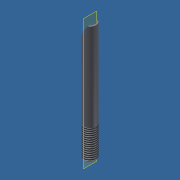
# Autodesk Inventor part: ESCAPAMENTO(16)
Saved by Autodesk Inventor 2012 SP1 (Build 160190100, 190)
## iProperties
Created: 2012-07-23
Part Number: ESCAPAMENTO(16)
Material: Carbon Steel
Document SubType Name: Modeling
Designer: bruno.silveira
Mass: 20.7136 g
Surface Area: 26.512 cm^2
Volume: 2.63197 cm^3
Density: 7.87 g/cm^3
Author: bruno.silveira
Autodesk Inventor part; units mm, degrees
ref_plane "YZ Plane" through (0, 0, 0) normal (1, 0, 0) x (0, 1, 0)
ref_plane "XZ Plane" through (0, 0, 0) normal (0, 1, 0) x (-1, 0, 0)
ref_plane "XY Plane" through (0, 0, 0) normal (0, 0, 1) x (1, 0, 0)
sketch "Sketch1" plane through (0, 0, 0) normal (0, 0, 1) x (1, 0, 0)
  circle A0 centre (0, 0) radius 3.9688
  dimension "d0" = 7.9375
  constraints: 1 centre point, 1 coincident
  measures "d0" diameter of A0
extrude "Extrusion1" add sketch "Sketch1" along normal blind 78
thread "Thread1" size "M8x1.25" class "6g" standard "ANSI Metric M Profile" length 20
sketch "Sketch2" plane through (0, 0, 78) normal (0, 0, 1) x (1, 0, 0)
  circle A0 centre (0, 0) radius 3.9687 projected
  constraints: 1 coincident
hole "Hole1" at (0, 0, 78) direction (0, 0, -1) diameter 6 depth 40 tip angle 118
sketch "Sketch3" plane through (0, 0, 0) normal (0, 1, 0) x (-1, 0, 0)
  line L0 (-3.9688, 78) -> (3.9688, 78) projected
  line L1 (-3.9688, 0) -> (3.9688, 0) projected
  line L2 (-1.8048, 78) -> (3.9688, 68)
  line L3 (3.9688, 0) -> (3.9688, 78) projected
  line L4 (-3.9688, 0) -> (-3.9688, 78) projected
  point P0 (0, 0)
  dimension "d12" = 30
  dimension "d13" = 10
  constraints: 2 end point, 2 point on line
  measures "d12" angle of L3 L2
  measures "d13" distance from line of L0 L2.end
extrude "Extrusion2" cut sketch "Sketch3" along normal mid plane 20 contours L0 L3 L2
chamfer "Chamfer1" distance 1 angle 45 1 edges at (-3.9688, 0, 0)
body "Solid1"
